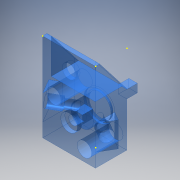
# Autodesk Inventor part: uppernozzle
Saved by Autodesk Inventor 2016 SP2 (Build 200236200, 236)
## iProperties
Created: 2017-01-26
Part Number: uppernozzle
Material: Water
Document SubType Name: Modeling
Designer: Teta
Density: 0.9983 g/cm^3
Appearance: Tropical Blue
Author: Teta
Autodesk Inventor part; units mm, degrees
ref_plane "YZ Plane" through (0, 0, 0) normal (1, 0, 0) x (0, 1, 0)
sketch "Sketch1" plane through (0, 0, 0) normal (0, 1, 0) x (-1, 0, 0)
  line L0 (0, 0) -> (25.5, 0)
  line L1 (25.5, 0) -> (25.5, -42.5)
  line L2 (25.5, -42.5) -> (0, -42.5)
  line L3 (0, -42.5) -> (0, 0)
  dimension "d0" = 25.5
  dimension "d1" = 42.5
  constraints: 8 end point, 2 parallel, 1 horizontal, 1 perpendicular
  measures "d0" distance of L1.end L2.end
  measures "d1" distance of L0.end L1.end
extrude "Extrusion1" add sketch "Sketch1" along normal blind 2
sketch "Sketch2" plane through (0, 2, 0) normal (0, 1, 0) x (1, 0, 0)
  line L0 (-25.5, 0) -> (0, 0) projected
  line L1 (-12.75, 0) -> (-2.25, 0)
  line L2 (-2.25, 0) -> (-23.25, 0)
  line L3 (-23.25, 0) -> (-23.25, 16.7)
  line L4 (-23.25, 16.7) -> (-2.25, 16.7)
  line L5 (-2.25, 16.7) -> (-2.25, 0)
  line L6 (-2.25, 0) -> (0, 0)
  line L7 (0, 0) -> (0, 19.3638)
  line L8 (0, 0) -> (0, 42.5) projected
  line L9 (0, 19.3638) -> (-25.5, 19.3638)
  line L10 (-25.5, 19.3638) -> (-25.5, 0)
  line L11 (-25.5, 0) -> (-23.25, 0)
  dimension "d4" = 10.5
  dimension "d5" = 21
  dimension "d6" = 16.7
  constraints: 20 end point, 4 perpendicular, 3 point on line, 1 collinear, 1 horizontal, 1 midpoint, 1 parallel
  measures "d4" distance of L1.start L1.end
  measures "d5" distance of L1.end L2.end
  measures "d6" distance of L2.end L3.end
extrude "Extrusion2" add sketch "Sketch2" along normal blind 13 contours L10 L9 L7 L0 L5 L4 L3
sketch "Sketch3" plane through (0, 0, 0) normal (1, 0, 0) x (0, 0, -1)
  line L0 (0, 2) -> (16.7, 2) projected
  line L1 (42.5, 0) -> (0, 0) projected
  line L2 (42.5, 0) -> (42.5, 2) projected
  line L3 (19.3638, 2) -> (42.5, 2) projected
  line L4 (19.3638, 2) -> (19.3638, 15) projected
  line L5 (0, 15) -> (19.3638, 15) projected
  line L6 (0, 0) -> (0, 15) projected
  line L7 (16.7, 2) -> (16.7, 15)
  line L8 (16.7, 15) -> (0, 2)
  line L9 (0, 0) -> (0, 15) projected
  line L10 (0, 2) -> (0, 15)
  line L11 (0, 15) -> (16.7, 15)
  constraints: 8 end point, 2 collinear, 1 point on line, 1 vertical
extrude "Extrusion3" cut sketch "Sketch3" against normal blind 130 contours L6 L5 L8
sketch "Sketch4" plane through (0, 2, 0) normal (0, 1, 0) x (1, 0, 0)
  line L0 (-23.25, 16.7) -> (-23.25, 0) projected
  line L1 (-23.25, 0) -> (-2.25, 0) projected
  line L2 (-2.25, 0) -> (-2.25, 16.7) projected
  line L3 (-2.25, 16.7) -> (-23.25, 16.7) projected
  circle A0 centre (-12.75, 8.35) radius 3.25
  point P0 (0, 0)
  dimension "d11" = 6.5
  constraints: 1 centre point
  measures "d11" diameter of A0
extrude "Extrusion4" cut sketch "Sketch4" against normal blind 130 contours A0
sketch "Sketch5" plane through (0, 2, 0) normal (0, 1, 0) x (1, 0, 0)
  line L0 (-25.5, 19.3638) -> (0, 19.3638) projected
  line L1 (0, 19.3638) -> (0, 42.5) projected
  line L2 (0, 42.5) -> (-25.5, 42.5) projected
  line L3 (-25.5, 42.5) -> (-25.5, 19.3638) projected
  point P0 (0, 0)
extrude "Extrusion5" add sketch "Sketch5" along normal blind 13
sketch "Sketch6" plane through (0, 15, 0) normal (0, 1, 0) x (1, 0, 0)
  point P0 (0, 0)
sketch "Sketch7" plane through (0, 15, 0) normal (0, 1, 0) x (1, 0, 0)
  line L0 (-25.5, 16.7) -> (-23.25, 16.7) projected
  line L1 (-23.25, 16.7) -> (-2.25, 16.7) projected
  line L2 (-2.25, 16.7) -> (0, 16.7) projected
  line L3 (0, 16.7) -> (0, 42.5) projected
  line L4 (0, 42.5) -> (-25.5, 42.5) projected
  line L5 (-25.5, 42.5) -> (-25.5, 16.7) projected
  circle A0 centre (-12.75, 29.6) radius 5.4
  point P0 (0, 0)
  dimension "d16" = 10.8
  constraints: 1 centre point
  measures "d16" diameter of A0
extrude "Extrusion6" cut sketch "Sketch7" against normal blind 8.8 contours A0
sketch "Sketch8" plane through (-12.75, 6.2, -29.6) normal (0, 1, 0) x (1, 0, 0)
  circle A0 centre (0, 0) radius 5.4 projected
  circle A1 centre (0, 0) radius 2.075
  point P0 (12.75, -29.6)
  dimension "d19" = 4.15
  constraints: 1 centre point, 1 coincident
  measures "d19" diameter of A1
extrude "Extrusion7" cut sketch "Sketch8" against normal blind 8.8 contours A1
sketch "Sketch9" plane through (0, 15, 0) normal (0, 1, 0) x (1, 0, 0)
  line L0 (-25.35, 42.2) -> (-0.15, 42.2)
  line L1 (-0.15, 42.2) -> (-0.15, 17)
  line L2 (-0.15, 17) -> (-25.35, 17)
  line L3 (-25.35, 17) -> (-25.35, 42.2)
  line L4 (-0.15, 17) -> (-4.15, 17)
  line L5 (-4.15, 17) -> (-4.15, 21)
  line L6 (-4.15, 21) -> (-0.15, 21)
  line L7 (-0.15, 21) -> (-0.15, 17)
  line L8 (-25.35, 42.2) -> (-21.35, 42.2)
  line L9 (-21.35, 42.2) -> (-21.35, 38.2)
  line L10 (-21.35, 38.2) -> (-25.35, 38.2)
  line L11 (-25.35, 38.2) -> (-25.35, 42.2)
  circle A0 centre (-12.75, 29.6) radius 5.4 projected
  line L12 (-25.5, 16.7) -> (-23.25, 16.7) projected
  line L13 (-23.25, 16.7) -> (-2.25, 16.7) projected
  line L14 (-2.25, 16.7) -> (0, 16.7) projected
  line L15 (0, 16.7) -> (0, 42.5) projected
  line L16 (0, 42.5) -> (-25.5, 42.5) projected
  line L17 (-25.5, 42.5) -> (-25.5, 16.7) construction
  line L18 (-25.35, 42.2) -> (-27.4299, 42.2)
  line L19 (-27.4299, 42.2) -> (-27.4299, -5.4814)
  line L20 (-27.4299, -5.4814) -> (-25.35, -5.4814)
  line L21 (-25.35, -5.4814) -> (-25.35, 42.2)
  line L22 (-25.35, 42.2) -> (-27.4299, 42.2)
  line L23 (-27.4299, 42.2) -> (-27.4299, 44.6012)
  line L24 (-27.4299, 44.6012) -> (-25.35, 44.6012)
  line L25 (-25.35, 44.6012) -> (-25.35, 42.2)
  line L26 (-27.4299, 44.6012) -> (1.4745, 44.6012)
  line L27 (1.4745, 44.6012) -> (1.4745, 42.2)
  line L28 (1.4745, 42.2) -> (-27.4299, 42.2)
  line L29 (-27.4299, 42.2) -> (-27.4299, 44.6012)
  line L30 (-0.15, 17) -> (3.4405, 17)
  line L31 (3.4405, 17) -> (3.4405, 44.8771)
  line L32 (3.4405, 44.8771) -> (-0.15, 44.8771)
  line L33 (-0.15, 44.8771) -> (-0.15, 17)
  line L34 (-0.15, 17) -> (3.4405, 17)
  line L35 (3.4405, 17) -> (3.4405, -4.7226)
  line L36 (3.4405, -4.7226) -> (-0.15, -4.7226)
  line L37 (-0.15, -4.7226) -> (-0.15, 17)
  point P0 (0, 0)
  dimension "d22" = 25.2
  dimension "d23" = 25.2
  dimension "d24" = 4
  dimension "d25" = 4
  dimension "d26" = 4
  dimension "d27" = 4
  constraints: 64 end point, 16 parallel, 8 horizontal, 8 perpendicular, 3 point on line
  measures "d22" distance of L1.end L2.end
  measures "d23" distance of L0.end L1.end
  measures "d24" distance of L5.end L6.end
  measures "d25" distance of L4.end L5.end
  measures "d26" distance of L9.end L10.end
  measures "d27" distance of L8.end L9.end
extrude "Extrusion8" add sketch "Sketch9" along normal blind 5 contours L25 L16 L33 L0 | L0 L9 L10 L3 | L3 L21 L20 L19 L18 | L25 L26 L33 L16 | L28 L15 L30 L1 | L33 L16 L15 L28 | L33 L26 L27 L28 L15 L16 | L1 L2 L5 L6 | L28 L27 L26 L33 L32 L31 L30 L15 | L30 L15 L14 L37 | L30 L35 L36 L37 L14 L15
sketch "Sketch10" plane through (0, 20, 0) normal (0, 1, 0) x (1, 0, 0)
  line L0 (-0.15, 42.2) -> (-0.15, 21) projected
  line L1 (-0.15, 21) -> (-4.15, 21) projected
  line L2 (-4.15, 21) -> (-4.15, 17) projected
  line L3 (-4.15, 17) -> (-0.15, 17) projected
  line L4 (-0.15, 17) -> (-0.15, -4.7226) projected
  line L5 (-0.15, -4.7226) -> (3.4405, -4.7226) projected
  line L6 (3.4405, -4.7226) -> (3.4405, 44.8771) projected
  line L7 (3.4405, 44.8771) -> (-0.15, 44.8771) projected
  line L8 (-0.15, 44.8771) -> (-0.15, 44.6012) projected
  line L9 (-0.15, 44.6012) -> (-25.35, 44.6012) projected
  line L10 (-25.35, 44.6012) -> (-25.35, 42.2) projected
  line L11 (-25.35, 42.2) -> (-27.4299, 42.2) projected
  line L12 (-27.4299, 42.2) -> (-27.4299, -5.4814) projected
  line L13 (-27.4299, -5.4814) -> (-25.35, -5.4814) projected
  line L14 (-25.35, -5.4814) -> (-25.35, 38.2) projected
  line L15 (-25.35, 38.2) -> (-21.35, 38.2) projected
  line L16 (-21.35, 38.2) -> (-21.35, 42.2) projected
  line L17 (-21.35, 42.2) -> (-0.15, 42.2) projected
  line L18 (-21.35, 42.2) -> (-21.35, 38.2) projected
  line L19 (-21.35, 38.2) -> (-25.35, 38.2)
  line L20 (-25.35, 38.2) -> (-25.35, 42.2)
  line L21 (-25.35, 42.2) -> (-21.35, 42.2)
  line L22 (-21.35, 42.2) -> (-21.35, 38.2)
  line L23 (-0.15, 42.2) -> (-0.15, 21) projected
  line L24 (-0.15, 21) -> (-4.15, 21)
  line L25 (-4.15, 21) -> (-4.15, 17)
  line L26 (-4.15, 17) -> (-0.15, 17)
  line L27 (-0.15, 17) -> (-0.15, 21)
  line L28 (-25.5, 42.2) -> (-25.35, 42.2) projected
  line L29 (-25.35, 42.2) -> (-25.35, 42.5) projected
  line L30 (-25.35, 42.5) -> (-25.5, 42.5) projected
  line L31 (-25.5, 42.5) -> (-25.5, 42.2) projected
  point P0 (0, 0)
  constraints: 16 end point, 4 parallel, 2 horizontal, 2 perpendicular
extrude "Extrusion9" cut sketch "Sketch10" against normal blind 1000 contours L17 L21 L10 L9 L8 L7 L6 L5 L4 L27 L0 | L20 L14 L13 L12 L11
sketch "Sketch11" plane through (0, 15, 0) normal (0, 1, 0) x (1, 0, 0)
  line L0 (-25.5, 42.2) -> (-25.35, 42.2) projected
  line L1 (-25.35, 42.2) -> (-25.35, 42.5) projected
  line L2 (-25.35, 42.5) -> (-25.5, 42.5) projected
  line L3 (-25.5, 42.5) -> (-25.5, 42.2) projected
  point P0 (0, 0)
extrude "Extrusion10" cut sketch "Sketch11" against normal blind 1000
sketch "Sketch12" plane through (0, 15, 0) normal (0, 1, 0) x (1, 0, 0)
  circle A0 centre (-20.0808, 22.2584) radius 2.625
  circle A1 centre (-20.0808, 22.2584) radius 2.625
  circle A2 centre (-5.4083, 36.9307) radius 2.625
  circle A3 centre (-12.75, 29.6) radius 5.5
  arc A4 (-25.35, 19) -> (-23.35, 17) centre (-23.35, 19) ccw
  line L0 (-4.15, 17) -> (-23.35, 17)
  line L1 (-4.15, 17) -> (-4.15, 21)
  line L2 (-4.15, 21) -> (-0.15, 21)
  line L3 (-0.15, 40.2) -> (-0.15, 21)
  arc A5 (-0.15, 40.2) -> (-2.15, 42.2) centre (-2.15, 40.2) ccw
  line L4 (-21.35, 42.2) -> (-2.15, 42.2)
  line L5 (-21.35, 42.2) -> (-21.35, 38.2)
  line L6 (-21.35, 38.2) -> (-25.35, 38.2)
  line L7 (-25.35, 19) -> (-25.35, 38.2)
  circle A6 centre (-12.75, 29.6) radius 2.075 projected
  circle A7 centre (-12.75, 29.6) radius 5.4 projected
  point P0 (0, 0)
  point P1 (-25.35, 42.2)
  constraints: 16 end point, 6 centre point, 4 point on circle
extrude "Extrusion11" cut sketch "Sketch12" against normal blind 1000 contours A0 | A2
sketch "Sketch13" plane through (0, 0, 0) normal (0, -1, 0) x (1, 0, 0)
  circle A0 centre (-5.4083, -36.9307) radius 2.625 projected
  circle A1 centre (-20.0808, -22.2584) radius 2.625 projected
  line L0 (-25.35, 0) -> (-25.35, -42.2) projected
  line L1 (-25.35, -42.2) -> (-0.15, -42.2) projected
  line L2 (-0.15, -42.2) -> (-0.15, 0) projected
  line L3 (-0.15, 0) -> (-25.35, 0) projected
  circle A2 centre (-12.75, -8.35) radius 3.25 projected
  circle A3 centre (-12.75, -29.6) radius 2.075 projected
  circle A4 centre (-20.0808, -22.2584) radius 3.45
  circle A5 centre (-5.4083, -36.9307) radius 3.45
  point P0 (0, 0)
  dimension "d36" = 6.9
  dimension "d37" = 6.9
  constraints: 2 centre point, 2 coincident
  measures "d36" diameter of A4
  measures "d37" diameter of A5
extrude "Extrusion12" cut sketch "Sketch13" against normal blind 1000 contours A4 | A5
sketch "Sketch14" plane through (0, 0, 0) normal (0, -1, 0) x (1, 0, 0)
  circle A0 centre (-20.0808, -22.2584) radius 3.45 projected
  circle A1 centre (-5.4083, -36.9307) radius 3.45 projected
  line L0 (-25.35, 0) -> (-25.35, -42.2) projected
  line L1 (-25.35, -42.2) -> (-0.15, -42.2) projected
  line L2 (-0.15, -42.2) -> (-0.15, 0) projected
  line L3 (-0.15, 0) -> (-25.35, 0) projected
  circle A2 centre (-12.75, -8.35) radius 3.25 projected
  circle A3 centre (-12.75, -29.6) radius 2.075 projected
  circle A4 centre (-12.75, -29.6) radius 4
  point P0 (0, 0)
  dimension "d40" = 8
  constraints: 1 centre point, 1 coincident
  measures "d40" diameter of A4
extrude "Extrusion13" cut sketch "Sketch14" against normal blind 2 contours A4
sketch "Sketch15" plane through (0, 15, 0) normal (0, 1, 0) x (1, 0, 0)
  circle A0 centre (-20.0808, 22.2584) radius 3.45 projected
  circle A1 centre (-5.4083, 36.9307) radius 3.45 projected
  circle A2 centre (-12.75, 29.6) radius 5.4 projected
  line L0 (-0.15, 16.7) -> (-0.15, 17) projected
  line L1 (-0.15, 17) -> (-4.15, 17) projected
  line L2 (-4.15, 17) -> (-4.15, 21) projected
  line L3 (-4.15, 21) -> (-0.15, 21) projected
  line L4 (-0.15, 21) -> (-0.15, 42.2) projected
  line L5 (-0.15, 42.2) -> (-21.35, 42.2) projected
  line L6 (-21.35, 42.2) -> (-21.35, 38.2) projected
  line L7 (-21.35, 38.2) -> (-25.35, 38.2) projected
  line L8 (-25.35, 38.2) -> (-25.35, 16.7) projected
  line L9 (-25.35, 16.7) -> (-23.25, 16.7) projected
  line L10 (-23.25, 16.7) -> (-2.25, 16.7) projected
  line L11 (-2.25, 16.7) -> (-0.15, 16.7) projected
  circle A3 centre (-12.75, 29.6) radius 6.95
  circle A4 centre (-12.75, 29.6) radius 6
  point P0 (0, 0)
  dimension "d43" = 13.9
  dimension "d44" = 12
  constraints: 2 centre point, 2 coincident
  measures "d43" diameter of A3
  measures "d44" diameter of A4
extrude "Extrusion14" cut sketch "Sketch15" against normal blind 1 contours A3 A0 | A0 A3 A1 | A3 A1 picked at (-17.6229, 24.6665) picked at (-7.8164, 34.4729)
sketch "Sketch16" plane through (-25.35, 20, -42.2) normal (-1, 0, 0) x (0, 0, 1)
  point P0 (42.2, -20)
ref_plane "Work Plane1" through (-25.35, 0, -29.725) normal (-0.866, -0.5, 0) x (0, 0, -1)
sketch "Sketch17" plane through (-25.35, 0, -29.725) normal (-0.866, -0.5, 0) x (0, 0, -1)
  line L0 (-29.725, 0) -> (12.475, 0) projected
  ellipse E0 centre (-0.125, 4.5679) end of major axis (1.95, 4.5679) minor radius 1.0375 projected
  ellipse E1 centre (-0.125, 6.3) end of major axis (-4.125, 6.3) minor radius 2 projected
  ellipse E2 centre (-0.125, -6.6904) end of major axis (5.275, -6.6904) minor radius 2.7 projected
  line L1 (-0.125, -6.6904) -> (-0.125, 6.3)
  line L2 (-0.125, 0) -> (3.875, 0)
  line L3 (3.875, 0) -> (-4.125, 0)
  line L4 (-4.125, 0) -> (-4.125, -8)
  line L5 (-4.125, -8) -> (3.875, -8)
  line L6 (3.875, -8) -> (3.875, 0)
  point P0 (-29.725, 12.675)
  dimension "d48" = 4
  dimension "d49" = 8
  dimension "d50" = 8
  constraints: 12 end point, 3 point on line, 2 parallel, 1 horizontal, 1 perpendicular, 1 vertical, 3 other
  measures "d48" distance of L2.start L2.end
  measures "d49" distance of L5.end L4.end
  measures "d50" distance of L4.end L3.end
extrude "Extrusion15" add sketch "Sketch17" against normal blind 4 contours L0 L1 E2 L4 | L0 L6 E2 L1 | E2 L6 L5 L4 picked at (-0.125, -6.6635)
sketch "Sketch18" plane through (-21.8859, 2, -29.725) normal (0.866, 0.5, 0) x (0, 0, -1)
  line L0 (3.875, 8) -> (-4.125, 8) projected
  line L1 (3.875, 6.9282) -> (-4.125, 6.9282) projected
  line L2 (3.875, 6.9282) -> (3.875, 8) projected
  line L3 (3.875, 8) -> (-4.125, 8) projected
  line L4 (-4.125, 8) -> (-4.125, 6.9282) projected
  point P0 (-29.725, -12.675)
extrude "Extrusion16" add sketch "Sketch18" along normal blind 1
ref_plane "Work Plane2" through (-12.75, 20, -42.2) normal (-1, 0, 0) x (0, 0, 1)
mirror "Mirror1" about plane through (-12.75, 20, -42.2) normal (-1, 0, 0) of "Extrusion15"
sketch "Sketch19" plane through (-0.15, 8, -33.6) normal (-0.866, 0.5, 0) x (0, 0, 1)
  line L0 (8, 0) -> (0, 0) projected
  line L1 (8, 1.0718) -> (8, 0) projected
  line L2 (0, 1.0718) -> (8, 1.0718) projected
  line L3 (0, 0) -> (0, 1.0718) projected
  point P0 (33.6, -6.8532)
extrude "Extrusion17" add sketch "Sketch19" along normal blind 1
sketch "Sketch20" plane through (3.85, 6.9282, -25.6) normal (0.866, -0.5, 0) x (0, 0, -1)
  point P0 (-25.6, -7.925)
sketch "Sketch21" plane through (3.85, 6.9282, -25.6) normal (0.866, -0.5, 0) x (0, 0, -1)
  line L0 (8, -8) -> (0, -8) projected
  line L1 (8, 0) -> (8, -8) projected
  line L2 (0, 0) -> (8, 0) projected
  line L3 (0, -8) -> (0, 0) projected
  line L4 (8, -8) -> (0, -8) projected
  line L5 (0, -8) -> (0, 0) projected
  circle A0 centre (4, -4) radius 2.75
  point P0 (-25.6, -7.925)
  dimension "d58" = 5.5
  constraints: 1 centre point
  measures "d58" diameter of A0
extrude "Extrusion18" cut sketch "Sketch21" against normal blind 6 contours A0
sketch "Sketch22" plane through (-3.3462, 6.4641, -29.6) normal (0.866, -0.5, 0) x (0, 0, -1)
  circle A0 centre (0, 0) radius 2.75 projected
  circle A1 centre (0, 0) radius 2
  point P0 (-29.6, -3.925)
  dimension "d61" = 4
  constraints: 1 centre point, 1 coincident
  measures "d61" diameter of A1
extrude "Extrusion19" cut sketch "Sketch22" against normal blind 6 contours A1
mirror "Mirror2" about plane through (-12.75, 20, -42.2) normal (-1, 0, 0) of "Extrusion18", "Extrusion19"
sketch "Sketch23" plane through (-25.35, 0, -33.6) normal (0, 0, -1) x (-1, 0, 0)
  line L0 (0, 0) -> (0, 9.2376) projected
  line L1 (4, 6.9282) -> (0, 0) projected
  line L2 (4, 6.9282) -> (0, 9.2376) projected
  point P0 (-25.35, 0)
extrude "Extrusion20" add sketch "Sketch23" along normal blind 2
sketch "Sketch24" plane through (-25.35, 0, -25.6) normal (0, 0, 1) x (1, 0, 0)
  line L0 (1.8212, 8.8457) -> (-3.375, 5.8457) projected
  line L1 (0, 9.2376) -> (0, 0) projected
  line L2 (-4, 6.9282) -> (0, 9.2376) projected
  line L3 (0, 0) -> (-4, 6.9282) projected
  point P0 (25.35, 0)
extrude "Extrusion21" add sketch "Sketch24" along normal blind 2
sketch "Sketch25" plane through (-0.15, 0, -25.6) normal (0, 0, 1) x (1, 0, 0)
  line L0 (0, 0) -> (0, 9.2376) projected
  line L1 (0, 0) -> (4, 6.9282) projected
  line L2 (4, 6.9282) -> (0, 9.2376) projected
  point P0 (0.15, 0)
extrude "Extrusion22" add sketch "Sketch25" along normal blind 2
sketch "Sketch26" plane through (-0.15, 0, -33.6) normal (0, 0, -1) x (-1, 0, 0)
  point P0 (-0.15, 0)
sketch "Sketch27" plane through (-0.15, 0, -33.6) normal (0, 0, -1) x (-1, 0, 0)
  line L0 (0, 9.2376) -> (0, 0) projected
  line L1 (-4, 6.9282) -> (0, 9.2376) projected
  line L2 (-4, 6.9282) -> (0, 0) projected
  point P0 (-0.15, 0)
extrude "Extrusion23" add sketch "Sketch27" along normal blind 2
sketch "Sketch28" plane through (0, 0, 0) normal (0, -1, 0) x (1, 0, 0)
  circle A0 centre (-12.75, -29.6) radius 4 projected
  circle A1 centre (-20.0808, -22.2584) radius 3.45 projected
  circle A2 centre (-5.4083, -36.9307) radius 3.45 projected
  line L0 (-25.35, 0) -> (-25.35, -23.6) projected
  line L1 (-25.35, -23.6) -> (-25.35, -35.6) projected
  line L2 (-25.35, -35.6) -> (-25.35, -42.2) projected
  line L3 (-25.35, -42.2) -> (-0.15, -42.2) projected
  line L4 (-0.15, -42.2) -> (-0.15, -35.6) projected
  line L5 (-0.15, -35.6) -> (-0.15, -23.6) projected
  line L6 (-0.15, -23.6) -> (-0.15, 0) projected
  line L7 (-0.15, 0) -> (-25.35, 0) projected
  circle A3 centre (-12.75, -8.35) radius 3.25 projected
  circle A4 centre (-12.75, -29.6) radius 2.075 projected
  point P0 (0, 0)
sketch "Sketch29" plane through (-12.75, 2, -29.6) normal (0, -1, 0) x (1, 0, 0)
  circle A0 centre (0, 0) radius 2.15
  point P0 (12.75, 29.6)
  dimension "d72" = 4.3
  constraints: 1 centre point
  measures "d72" diameter of A0
extrude "Extrusion24" cut sketch "Sketch29" against normal blind 10
body "Solid1"
